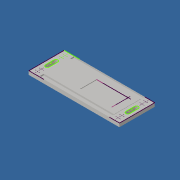
# Autodesk Inventor part: Button Fixture Base
Saved by Autodesk Inventor 2016 (Build 200138000, 138)
## iProperties
Created: 2016-07-07
Part Number: Button Fixture Base
Material: Generic
Document SubType Name: Modeling
Designer: Sam Clay
Density: 1 g/cm^3
Appearance: Default
Author: Sam Clay
Autodesk Inventor part; units mm, degrees
ref_plane "YZ Plane" through (0, 0, 0) normal (1, 0, 0) x (0, 1, 0)
ref_plane "XZ Plane" through (0, 0, 0) normal (0, 1, 0) x (-1, 0, 0)
ref_plane "XY Plane" through (0, 0, 0) normal (0, 0, 1) x (1, 0, 0)
sketch "Sketch1" plane through (0, 0, 0) normal (0, 1, 0) x (-1, 0, 0)
  line L0 (0, 0) -> (355.6, 0)
  line L1 (355.6, 0) -> (355.6, 177.8)
  line L2 (355.6, 177.8) -> (0, 177.8)
  line L3 (0, 177.8) -> (0, 0)
  line L4 (355.6, 0) -> (406.4, 0)
  line L5 (406.4, 0) -> (406.4, 177.8)
  line L6 (406.4, 177.8) -> (355.6, 177.8)
  line L7 (355.6, 177.8) -> (355.6, 0)
  line L8 (0, 0) -> (-50.8, 0)
  line L9 (-50.8, 0) -> (-50.8, 177.8)
  line L10 (-50.8, 177.8) -> (0, 177.8)
  line L11 (0, 177.8) -> (0, 0)
  dimension "d0" = 355.6
  dimension "d1" = 177.8
  dimension "d2" = 50.8
  dimension "d3" = 50.8
  constraints: 24 end point, 6 parallel, 3 horizontal, 3 perpendicular, 2 point on line
  measures "d0" distance of L2.end L1.end
  measures "d1" distance of L1.end L0.end
  measures "d2" distance of L6.end L5.end
  measures "d3" distance of L9.end L10.end
extrude "Extrusion1" add sketch "Sketch1" along normal blind 19.05 contours L3 L2 L1 L0
extrude "Extrusion2" add sketch "Sketch1" along normal blind 17.78 contours L8 L9 L10 L3 | L1 L6 L5 L4
sketch "Sketch2" plane through (0, 19.05, 0) normal (0, 1, 0) x (1, 0, 0)
  line L0 (-355.6, 0) -> (-355.6, -177.8) projected
  line L1 (0, 0) -> (-355.6, 0)
  line L2 (-355.6, 0) -> (-355.6, -0.254)
  line L3 (-355.6, -0.254) -> (0, -0.254)
  line L4 (0, -0.254) -> (0, 0)
  line L5 (0, -0.254) -> (-355.6, -0.254)
  line L6 (-355.6, -0.254) -> (-355.6, -20.066)
  line L7 (-355.6, -20.066) -> (0, -20.066)
  line L8 (0, -20.066) -> (0, -0.254)
  line L9 (0, -20.066) -> (-355.6, -20.066)
  line L10 (-355.6, -20.066) -> (-355.6, -45.466)
  line L11 (-355.6, -45.466) -> (0, -45.466)
  line L12 (0, -45.466) -> (0, -20.066)
  line L13 (0, -45.466) -> (-355.6, -45.466)
  line L14 (-355.6, -45.466) -> (-355.6, -128.016)
  line L15 (-355.6, -128.016) -> (0, -128.016)
  line L16 (0, -128.016) -> (0, -45.466)
  line L17 (0, -128.016) -> (-355.6, -128.016)
  line L18 (-355.6, -128.016) -> (-355.6, -153.416)
  line L19 (-355.6, -153.416) -> (0, -153.416)
  line L20 (0, -153.416) -> (0, -128.016)
  line L21 (0, -153.416) -> (-355.6, -153.416)
  line L22 (-355.6, -153.416) -> (-355.6, -173.228)
  line L23 (-355.6, -173.228) -> (0, -173.228)
  line L24 (0, -173.228) -> (0, -153.416)
  line L25 (0, -173.228) -> (-355.6, -173.228)
  line L26 (-355.6, -173.228) -> (-355.6, -176.403)
  line L27 (-355.6, -176.403) -> (0, -176.403)
  line L28 (0, -176.403) -> (0, -173.228)
  line L29 (0, -177.8) -> (0, 0) projected
  line L30 (0, 0) -> (-38.1, 0)
  line L31 (-38.1, 0) -> (-38.1, -128.016)
  line L32 (-38.1, -128.016) -> (0, -128.016)
  line L33 (0, -128.016) -> (0, 0)
  circle A0 centre (-41.6783, -48.641) radius 8.89
  line L34 (-38.1, -45.466) -> (-196.85, -45.466)
  line L35 (-196.85, -45.466) -> (-196.85, -128.016)
  line L36 (-196.85, -128.016) -> (-38.1, -128.016)
  line L37 (-38.1, -128.016) -> (-38.1, -45.466)
  dimension "d8" = 0.254
  dimension "d9" = 19.812
  dimension "d10" = 25.4
  dimension "d11" = 82.55
  dimension "d12" = 25.4
  dimension "d13" = 19.812
  dimension "d14" = 3.175
  dimension "d15" = 38.1
  dimension "d16" = 17.78
  dimension "d21" = 3.175
  dimension "d49" = 158.75
  constraints: 72 end point, 18 parallel, 11 point on line, 9 horizontal, 9 perpendicular, 1 centre point
  measures "d8" distance of L2.end L1.end
  measures "d9" distance of L6.end L5.end
  measures "d10" distance of L10.end L9.end
  measures "d11" distance of L14.end L13.end
  measures "d12" distance of L18.end L17.end
  measures "d13" distance of L22.end L21.end
  measures "d14" distance of L26.end L25.end
  measures "d15" distance of L32.end L31.end
  measures "d16" diameter of A0
  measures "d21" distance from line of L13 A0.centre
  measures "d49" distance of L36.end L35.end
extrude "Extrusion3" cut sketch "Sketch2" against normal blind 7.62 contours L3 L31 L7 L0 | L3 L8 L7 L31 | L19 L24 L23 L0
extrude "Extrusion4" cut sketch "Sketch2" against normal blind 3.175 contours L11 A0 L31 L15 L35 | A0 L11 L31 | L31 L11 A0 | L11 L31 A0 | L11 A0 L31
sketch "Sketch3" plane through (0, 19.05, 0) normal (0, 1, 0) x (1, 0, 0)
  line L0 (50.8, -177.8) -> (50.8, 0)
  line L1 (50.8, 0) -> (0, 0)
  line L2 (0, -177.8) -> (50.8, -177.8)
  line L3 (-406.4, 0) -> (-406.4, -177.8)
  line L4 (-330.2, 0) -> (-406.4, 0)
  line L5 (-406.4, -177.8) -> (-330.2, -177.8)
  line L6 (-381, -66.675) -> (-381, -111.125) construction
  line L7 (-390.525, -66.675) -> (-390.525, -111.125)
  line L8 (-371.475, -111.125) -> (-371.475, -66.675)
  arc A0 (-371.475, -66.675) -> (-390.525, -66.675) centre (-381, -66.675) ccw
  arc A1 (-390.525, -111.125) -> (-371.475, -111.125) centre (-381, -111.125) ccw
  line L9 (25.4, -66.675) -> (25.4, -111.125) construction
  line L10 (15.875, -66.675) -> (15.875, -111.125)
  line L11 (34.925, -111.125) -> (34.925, -66.675)
  arc A2 (34.925, -66.675) -> (15.875, -66.675) centre (25.4, -66.675) ccw
  arc A3 (15.875, -111.125) -> (34.925, -111.125) centre (25.4, -111.125) ccw
  line L12 (-165.1, -45.466) -> (-24.582, -45.466)
  line L13 (-38.1, -37.6081) -> (-38.1, -108.845)
  line L14 (-406.4, -177.8) -> (-355.6, -177.8) projected
  line L15 (0, -177.8) -> (50.8, -177.8) projected
  line L16 (50.8, 0) -> (0, 0) projected
  line L17 (50.8, -177.8) -> (50.8, 0) projected
  line L18 (-406.4, 0) -> (-406.4, -177.8) projected
  line L19 (-196.85, -45.466) -> (-49.982, -45.466) projected
  line L20 (-38.1, -56.7791) -> (-38.1, -128.016) projected
  point P0 (-38.1, -45.466)
  point P1 (25.4, -19.05)
  point P2 (25.4, -38.1)
  point P3 (25.4, -158.75)
  point P4 (25.4, -139.7)
  point P5 (-381, -19.05)
  point P6 (-381, -38.1)
  point P7 (-381, -158.75)
  point P8 (-381, -139.7)
  point P9 (-381, -88.9)
  point P10 (25.4, -88.9)
  dimension "d22" = 25.4
  dimension "d23" = 19.05
  dimension "d24" = 19.05
  dimension "d25" = 25.4
  dimension "d26" = 19.05
  dimension "d27" = 19.05
  dimension "d28" = 25.4
  dimension "d29" = 25.4
  dimension "d30" = 25.4
  dimension "d31" = 19.05
  dimension "d33" = 19.05
  dimension "d34" = 19.05
  dimension "d35" = 19.05
  dimension "d36" = 25.4
  dimension "d37" = 25.4
  dimension "d38" = 25.4
  dimension "d39" = 44.45
  dimension "d40" = 19.05
  dimension "d43" = 44.45
  dimension "d44" = 19.05
  constraints: 32 end point, 8 point on circle, 8 tangent, 7 collinear, 4 centre point, 2 midpoint, 2 parallel, 2 point on line, 2 vertical
  measures "d22" distance from line of L0 point (25.4, -19.05)
  measures "d23" distance from line of L1 point (25.4, -19.05)
  measures "d24" distance from line of L2 point (25.4, -158.75)
  measures "d25" distance from line of L0 point (25.4, -158.75)
  measures "d26" distance of point (25.4, -38.1) point (25.4, -19.05)
  measures "d27" distance of point (25.4, -139.7) point (25.4, -158.75)
  measures "d28" distance from line of L0 point (25.4, -139.7)
  measures "d29" distance from line of L0 point (25.4, -38.1)
  measures "d30" distance from line of L3 point (-381, -19.05)
  measures "d31" distance from line of L4 point (-381, -19.05)
  measures "d33" distance of point (-381, -19.05) point (-381, -38.1)
  measures "d34" distance of point (-381, -158.75) point (-381, -139.7)
  measures "d35" distance from line of L5 point (-381, -158.75)
  measures "d36" distance from line of L3 point (-381, -38.1)
  measures "d37" distance from line of L3 point (-381, -139.7)
  measures "d38" distance from line of L3 point (-381, -158.75)
  measures "d39" distance of L6.start L6.end
  measures "d40" diameter of A1
  measures "d43" distance of L9.start L9.end
  measures "d44" diameter of A3
extrude "Extrusion5" cut sketch "Sketch3" against normal through all
equation "\"d24\" = d23"
equation "\"d25\" = d22"
equation "\"d26\" = d23"
equation "\"d27\" = d26"
equation "\"d28\" = d22"
equation "\"d29\" = d22"
equation "\"d30\" = d22"
equation "\"d31\" = d23"
equation "\"d33\" = d31"
equation "\"d34\" = d31"
equation "\"d35\" = d31"
equation "\"d36\" = d22"
equation "\"d37\" = d22"
equation "\"d38\" = d22"
equation "\"d39\" = d43"
equation "\"d40\" = d44"
body "Solid1"
